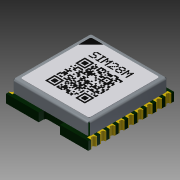
# Autodesk Inventor part: SIM28M
Saved by Autodesk Inventor 2015 SP1 (Build 190203100, 203)
## iProperties
Created: 2015-01-28
Part Number: SIM28M
Material: Типовые
Document SubType Name: Modeling
Designer: Danil
Density: 1 g/cm^3
Appearance: Цинк
Author: Danil
Autodesk Inventor part; units mm, degrees
(part 1 of 2)
ref_plane "YZ Plane" through (0, 0, 0) normal (1, 0, 0) x (0, 1, 0)
sketch "Эскиз1" plane through (0, 0, 0) normal (0, 0, 1) x (1, 0, 0)
  line L0 (4.85, -5.05) -> (-4.85, 5.05) construction
  line L1 (-4.85, -5.05) -> (4.85, 5.05) construction
  line L2 (-1.5, 5.05) -> (-2, 5.05)
  line L3 (1, 4.5) -> (1, 5.05)
  line L4 (-1.5, 5.05) -> (-1.5, 4.5)
  line L5 (-1.25, 4.25) -> (0.75, 4.25)
  line L6 (-4.85, 5.05) -> (-3.85, 5.05)
  line L7 (1, 5.05) -> (1.5, 5.05)
  line L8 (1.5, -5.05) -> (1.5, -4.5)
  line L9 (1.25, -4.25) -> (0, -4.25)
  line L10 (-1, -5.05) -> (-1, -4.5)
  line L11 (-0.75, -4.25) -> (0, -4.25)
  line L12 (4.85, -5.05) -> (1.5, -5.05)
  line L13 (-1, -5.05) -> (-4.85, -5.05)
  arc A0 (0.75, 4.25) -> (1, 4.5) centre (0.75, 4.5) ccw
  arc A1 (-1.5, 4.5) -> (-1.25, 4.25) centre (-1.25, 4.5) ccw
  arc A2 (1.5, -4.5) -> (1.25, -4.25) centre (1.25, -4.5) ccw
  arc A3 (-0.75, -4.25) -> (-1, -4.5) centre (-0.75, -4.5) ccw
  line L14 (4.85, -5.05) -> (1.5, -5.05)
  line L15 (-4.85, 5.05) -> (-1.5, 5.05)
  line L16 (1, 5.05) -> (4.85, 5.05)
  line L17 (-1, -5.05) -> (-4.85, -5.05)
  line L18 (-3.85, 5.05) -> (-1.5, 5.05)
  line L19 (1.5, 5.05) -> (4.85, 5.05)
  line L20 (-1.7057, -5.05) -> (-1, -5.05)
  line L21 (1.5, -5.05) -> (2.7193, -5.05)
  line L22 (-4.85, 1.8825) -> (-4.85, 3.4137)
  arc A4 (-4.85, 4.14) -> (-4.85, 4.66) centre (-4.85, 4.4) ccw
  line L23 (-4.85, 5.05) -> (-4.85, 4.66)
  arc A5 (-4.85, 3.04) -> (-4.85, 3.56) centre (-4.85, 3.3) ccw
  arc A6 (-4.85, 1.94) -> (-4.85, 2.46) centre (-4.85, 2.2) ccw
  arc A7 (-4.85, 0.84) -> (-4.85, 1.36) centre (-4.85, 1.1) ccw
  arc A8 (-4.85, -0.26) -> (-4.85, 0.26) centre (-4.85, 0) ccw
  arc A9 (-4.85, -1.36) -> (-4.85, -0.84) centre (-4.85, -1.1) ccw
  arc A10 (-4.85, -2.46) -> (-4.85, -1.94) centre (-4.85, -2.2) ccw
  arc A11 (-4.85, -3.56) -> (-4.85, -3.04) centre (-4.85, -3.3) ccw
  arc A12 (-4.85, -4.66) -> (-4.85, -4.14) centre (-4.85, -4.4) ccw
  arc A13 (4.85, 4.66) -> (4.85, 4.14) centre (4.85, 4.4) ccw
  arc A14 (4.85, 3.56) -> (4.85, 3.04) centre (4.85, 3.3) ccw
  arc A15 (4.85, 2.46) -> (4.85, 1.94) centre (4.85, 2.2) ccw
  arc A16 (4.85, 1.36) -> (4.85, 0.84) centre (4.85, 1.1) ccw
  arc A17 (4.85, 0.26) -> (4.85, -0.26) centre (4.85, 0) ccw
  arc A18 (4.85, -0.84) -> (4.85, -1.36) centre (4.85, -1.1) ccw
  arc A19 (4.85, -1.94) -> (4.85, -2.46) centre (4.85, -2.2) ccw
  arc A20 (4.85, -3.04) -> (4.85, -3.56) centre (4.85, -3.3) ccw
  arc A21 (4.85, -4.14) -> (4.85, -4.66) centre (4.85, -4.4) ccw
  line L24 (4.85, 5.05) -> (4.85, 4.66)
  line L25 (4.85, 4.14) -> (4.85, 3.56)
  line L26 (4.85, 3.04) -> (4.85, 2.46)
  line L27 (4.85, 1.94) -> (4.85, 1.36)
  line L28 (4.85, 0.84) -> (4.85, 0.26)
  line L29 (4.85, -0.26) -> (4.85, -0.84)
  line L30 (4.85, -1.36) -> (4.85, -1.94)
  line L31 (4.85, -2.46) -> (4.85, -3.04)
  line L32 (4.85, -3.56) -> (4.85, -4.14)
  line L33 (4.85, -4.66) -> (4.85, -5.05)
  line L34 (-4.85, -4.66) -> (-4.85, -5.05)
  line L35 (-4.85, -3.56) -> (-4.85, -4.14)
  line L36 (-4.85, -2.46) -> (-4.85, -3.04)
  line L37 (-4.85, -1.36) -> (-4.85, -1.94)
  line L38 (-4.85, -0.26) -> (-4.85, -0.84)
  line L39 (-4.85, 0.84) -> (-4.85, 0.26)
  line L40 (-4.85, 1.94) -> (-4.85, 1.36)
  line L41 (-4.85, 4.14) -> (-4.85, 3.56)
  line L42 (-4.85, 3.04) -> (-4.85, 2.46)
  point P0 (0, 0)
  point P1 (-4.85, -1.1)
  point P2 (4.85, -1.1)
  dimension "d497" = 1.1
  dimension "d93" = 9.7
  dimension "d98" = 0.25
  dimension "d148" = 0.26
  dimension "d149" = 0.26
  dimension "d150" = 0.26
  dimension "d151" = 0.26
  dimension "d152" = 0.26
  dimension "d153" = 0.26
  dimension "d154" = 0.26
  dimension "d155" = 0.26
  dimension "d156" = 0.26
  dimension "d157" = 0.26
  dimension "d158" = 0.26
  dimension "d159" = 0.26
  dimension "d160" = 0.26
  dimension "d161" = 0.26
  dimension "d162" = 0.26
  dimension "d163" = 0.26
  dimension "d164" = 0.26
  dimension "d165" = 0.26
  constraints: 86 end point, 44 point on circle, 22 centre point, 20 vertical, 12 parallel, 10 perpendicular, 8 tangent, 5 horizontal, 5 point on line, 3 equal radius, 2 coincident, 2 midpoint
  measures "d93" distance of L1.end L0.end
  measures "d98" radius of A0
  measures "d148" radius of A4
  measures "d149" radius of A5
  measures "d150" radius of A6
  measures "d151" radius of A7
  measures "d152" radius of A8
  measures "d153" radius of A9
  measures "d154" radius of A10
  measures "d155" radius of A11
  measures "d156" radius of A12
  measures "d157" radius of A13
  measures "d158" radius of A14
  measures "d159" radius of A15
  measures "d160" radius of A16
  measures "d161" radius of A17
  measures "d162" radius of A18
  measures "d163" radius of A19
  measures "d164" radius of A20
  measures "d165" radius of A21
extrude "Выдавливание2" add sketch "Эскиз1" along normal blind 1 contours L4 A1 L5 A0 L3 L7 L16 L24 A13 L25 A14 L26 A15 L27 A16 L28 A17 L29 A18 L30 A19 L31 A20 L32 A21 L33 L12 L8 A2 L9 L11 A3 L10 L13 L34 A12 L35 A11 L36 A10 L37 A9 L38 A8 L39 A7 L40 L22 A6 A5 L41 A4 L23 L6 L15 L2
sketch "Эскиз4" plane through (0, 0, 0) normal (0, 0, 1) x (1, 0, 0)
  arc A0 (-4.86, 4.15) -> (-4.86, 4.65) centre (-4.86, 4.4) ccw
  line L0 (-4.86, 4.4) -> (-4.86, 4.65) construction
  line L1 (-4.86, 4.4) -> (-4.61, 4.4) construction
  line L2 (-4.86, 4.4) -> (-4.86, 4.15) construction
  line L3 (-4.86, 4.65) -> (-4.86, 4.75)
  line L4 (-4.86, 4.65) -> (-4.76, 4.65) construction
  line L5 (-4.86, 4.75) -> (-4.41, 4.75)
  line L6 (-4.41, 4.75) -> (-4.41, 4.05)
  line L7 (-4.41, 4.05) -> (-4.86, 4.05)
  line L8 (-4.86, 4.05) -> (-4.86, 4.15)
  arc A1 (4.86, 4.65) -> (4.86, 4.15) centre (4.86, 4.4) ccw
  line L9 (4.86, 4.4) -> (4.86, 4.65) construction
  line L10 (4.86, 4.4) -> (5.11, 4.4) construction
  line L11 (4.86, 4.4) -> (4.86, 4.15) construction
  line L12 (4.86, 4.65) -> (4.86, 4.75)
  line L13 (4.86, 4.75) -> (4.41, 4.75)
  line L14 (4.41, 4.75) -> (4.41, 4.05)
  line L15 (4.41, 4.05) -> (4.86, 4.05)
  line L16 (4.86, 4.05) -> (4.86, 4.15)
  line L17 (4.86, 3.3) -> (4.86, 3.55) construction
  arc A2 (4.86, 3.55) -> (4.86, 3.05) centre (4.86, 3.3) ccw
  line L18 (4.86, 3.55) -> (4.86, 3.65)
  line L19 (4.86, 3.65) -> (4.41, 3.65)
  line L20 (4.41, 3.65) -> (4.41, 2.95)
  line L21 (4.41, 2.95) -> (4.86, 2.95)
  line L22 (4.86, 2.95) -> (4.86, 3.05)
  line L23 (4.86, 1.85) -> (4.86, 1.95)
  line L24 (4.41, 2.55) -> (4.41, 1.85)
  line L25 (4.86, 2.2) -> (4.86, 2.45) construction
  arc A3 (4.86, 2.45) -> (4.86, 1.95) centre (4.86, 2.2) ccw
  line L26 (4.86, 2.45) -> (4.86, 2.55)
  line L27 (4.86, 2.55) -> (4.41, 2.55)
  line L28 (4.41, 1.85) -> (4.86, 1.85)
  line L29 (4.86, 0.75) -> (4.86, 0.85)
  line L30 (4.41, 1.45) -> (4.41, 0.75)
  line L31 (4.86, 1.1) -> (4.86, 1.35) construction
  arc A4 (4.86, 1.35) -> (4.86, 0.85) centre (4.86, 1.1) ccw
  line L32 (4.86, 1.35) -> (4.86, 1.45)
  line L33 (4.86, 1.45) -> (4.41, 1.45)
  line L34 (4.41, 0.75) -> (4.86, 0.75)
  line L35 (4.86, -0.35) -> (4.86, -0.25)
  line L36 (4.41, 0.35) -> (4.41, -0.35)
  line L37 (4.86, 0) -> (4.86, 0.25) construction
  arc A5 (4.86, 0.25) -> (4.86, -0.25) centre (4.86, 0) ccw
  line L38 (4.86, 0.25) -> (4.86, 0.35)
  line L39 (4.86, 0.35) -> (4.41, 0.35)
  line L40 (4.41, -0.35) -> (4.86, -0.35)
  line L41 (4.86, -1.45) -> (4.86, -1.35)
  line L42 (4.41, -0.75) -> (4.41, -1.45)
  line L43 (4.86, -1.1) -> (4.86, -0.85) construction
  arc A6 (4.86, -0.85) -> (4.86, -1.35) centre (4.86, -1.1) ccw
  line L44 (4.86, -0.85) -> (4.86, -0.75)
  line L45 (4.86, -0.75) -> (4.41, -0.75)
  line L46 (4.41, -1.45) -> (4.86, -1.45)
  line L47 (4.86, -2.55) -> (4.86, -2.45)
  line L48 (4.41, -1.85) -> (4.41, -2.55)
  line L49 (4.86, -2.2) -> (4.86, -1.95) construction
  arc A7 (4.86, -1.95) -> (4.86, -2.45) centre (4.86, -2.2) ccw
  line L50 (4.86, -1.95) -> (4.86, -1.85)
  line L51 (4.86, -1.85) -> (4.41, -1.85)
  line L52 (4.41, -2.55) -> (4.86, -2.55)
  line L53 (4.86, -3.65) -> (4.86, -3.55)
  line L54 (4.41, -2.95) -> (4.41, -3.65)
  line L55 (4.86, -3.3) -> (4.86, -3.05) construction
  arc A8 (4.86, -3.05) -> (4.86, -3.55) centre (4.86, -3.3) ccw
  line L56 (4.86, -3.05) -> (4.86, -2.95)
  line L57 (4.86, -2.95) -> (4.41, -2.95)
  line L58 (4.41, -3.65) -> (4.86, -3.65)
  line L59 (4.86, -4.75) -> (4.86, -4.65)
  line L60 (4.41, -4.05) -> (4.41, -4.75)
  line L61 (4.86, -4.4) -> (4.86, -4.15) construction
  arc A9 (4.86, -4.15) -> (4.86, -4.65) centre (4.86, -4.4) ccw
  line L62 (4.86, -4.15) -> (4.86, -4.05)
  line L63 (4.86, -4.05) -> (4.41, -4.05)
  line L64 (4.41, -4.75) -> (4.86, -4.75)
  arc A10 (-4.86, 3.05) -> (-4.86, 3.55) centre (-4.86, 3.3) ccw
  line L65 (-4.86, 3.3) -> (-4.61, 3.3) construction
  line L66 (-4.86, 3.65) -> (-4.41, 3.65)
  line L67 (-4.41, 3.65) -> (-4.41, 2.95)
  line L68 (-4.41, 2.95) -> (-4.86, 2.95)
  line L69 (-4.86, 3.55) -> (-4.86, 3.65)
  line L70 (-4.86, 2.95) -> (-4.86, 3.05)
  line L71 (-4.86, 2.55) -> (-4.41, 2.55)
  line L72 (-4.86, 2.2) -> (-4.61, 2.2) construction
  arc A11 (-4.86, 1.95) -> (-4.86, 2.45) centre (-4.86, 2.2) ccw
  line L73 (-4.41, 1.85) -> (-4.86, 1.85)
  line L74 (-4.41, 2.55) -> (-4.41, 1.85)
  line L75 (-4.86, 2.45) -> (-4.86, 2.55)
  line L76 (-4.86, 1.85) -> (-4.86, 1.95)
  line L77 (-4.86, 1.45) -> (-4.41, 1.45)
  line L78 (-4.86, 1.1) -> (-4.61, 1.1) construction
  arc A12 (-4.86, 0.85) -> (-4.86, 1.35) centre (-4.86, 1.1) ccw
  line L79 (-4.41, 0.75) -> (-4.86, 0.75)
  line L80 (-4.41, 1.45) -> (-4.41, 0.75)
  line L81 (-4.86, 1.35) -> (-4.86, 1.45)
  line L82 (-4.86, 0.75) -> (-4.86, 0.85)
  line L83 (-4.86, 0.35) -> (-4.41, 0.35)
  line L84 (-4.86, 0) -> (-4.61, 0) construction
  arc A13 (-4.86, -0.25) -> (-4.86, 0.25) centre (-4.86, 0) ccw
  line L85 (-4.41, -0.35) -> (-4.86, -0.35)
  line L86 (-4.41, 0.35) -> (-4.41, -0.35)
  line L87 (-4.86, 0.25) -> (-4.86, 0.35)
  line L88 (-4.86, -0.35) -> (-4.86, -0.25)
  line L89 (-4.86, -0.75) -> (-4.41, -0.75)
  line L90 (-4.86, -1.1) -> (-4.61, -1.1) construction
  arc A14 (-4.86, -1.35) -> (-4.86, -0.85) centre (-4.86, -1.1) ccw
  line L91 (-4.41, -1.45) -> (-4.86, -1.45)
  line L92 (-4.41, -0.75) -> (-4.41, -1.45)
  line L93 (-4.86, -0.85) -> (-4.86, -0.75)
  line L94 (-4.86, -1.45) -> (-4.86, -1.35)
  line L95 (-4.86, -1.85) -> (-4.41, -1.85)
  line L96 (-4.86, -2.2) -> (-4.61, -2.2) construction
  arc A15 (-4.86, -2.45) -> (-4.86, -1.95) centre (-4.86, -2.2) ccw
  line L97 (-4.41, -2.55) -> (-4.86, -2.55)
  line L98 (-4.41, -1.85) -> (-4.41, -2.55)
  line L99 (-4.86, -1.95) -> (-4.86, -1.85)
  line L100 (-4.86, -2.55) -> (-4.86, -2.45)
  line L101 (-4.86, -2.95) -> (-4.41, -2.95)
  line L102 (-4.86, -3.3) -> (-4.61, -3.3) construction
  arc A16 (-4.86, -3.55) -> (-4.86, -3.05) centre (-4.86, -3.3) ccw
  line L103 (-4.41, -3.65) -> (-4.86, -3.65)
  line L104 (-4.41, -2.95) -> (-4.41, -3.65)
  line L105 (-4.86, -3.05) -> (-4.86, -2.95)
  line L106 (-4.86, -3.65) -> (-4.86, -3.55)
  line L107 (-4.86, -4.05) -> (-4.41, -4.05)
  line L108 (-4.86, -4.4) -> (-4.61, -4.4) construction
  arc A17 (-4.86, -4.65) -> (-4.86, -4.15) centre (-4.86, -4.4) ccw
  line L109 (-4.41, -4.75) -> (-4.86, -4.75)
  line L110 (-4.41, -4.05) -> (-4.41, -4.75)
  line L111 (-4.86, -4.15) -> (-4.86, -4.05)
  line L112 (-4.86, -4.75) -> (-4.86, -4.65)
  point P0 (-4.86, 0)
  point P1 (-4.86, -2.2)
  point P2 (-4.86, -3.3)
  point P3 (4.86, -2.2)
  point P4 (4.86, -3.3)
  point P5 (-4.86, -4.4)
  dimension "d354" = 0.25
  dimension "d355" = 90
  dimension "d356" = 180
  dimension "d357" = 0.1
  dimension "d358" = 90
  dimension "d359" = 0.45
  dimension "d360" = 0.7
  dimension "d361" = 0.25
  dimension "d362" = 90
  dimension "d363" = 180
  dimension "d364" = 0.1
  dimension "d365" = 0.45
  dimension "d366" = 0.7
  dimension "d367" = 0.25
  dimension "d368" = 0.1
  dimension "d369" = 0.45
  dimension "d370" = 0.7
  dimension "d371" = 0.25
  dimension "d372" = 0.1
  dimension "d373" = 0.45
  dimension "d374" = 0.7
  dimension "d375" = 0.25
  dimension "d376" = 0.1
  dimension "d377" = 0.45
  dimension "d378" = 0.7
  dimension "d379" = 0.25
  dimension "d380" = 0.1
  dimension "d381" = 0.45
  dimension "d382" = 0.7
  dimension "d383" = 0.25
  dimension "d384" = 0.1
  dimension "d385" = 0.45
  dimension "d386" = 0.7
  dimension "d387" = 0.25
  dimension "d388" = 0.1
  dimension "d389" = 0.45
  dimension "d390" = 0.7
  dimension "d391" = 0.25
  dimension "d392" = 0.1
  dimension "d393" = 0.45
  dimension "d394" = 0.7
  dimension "d395" = 0.25
  dimension "d396" = 0.1
  dimension "d397" = 0.45
  dimension "d398" = 0.7
  dimension "d399" = 0.25
  dimension "d400" = 0.1
  dimension "d401" = 0.45
  dimension "d402" = 0.7
  dimension "d403" = 0.25
  dimension "d404" = 0.1
  dimension "d405" = 0.45
  dimension "d406" = 0.7
  dimension "d407" = 0.25
  dimension "d408" = 0.1
  dimension "d409" = 0.45
  dimension "d410" = 0.7
  dimension "d411" = 0.25
  dimension "d412" = 0.1
  dimension "d413" = 0.45
  dimension "d414" = 0.7
  dimension "d415" = 0.25
  dimension "d416" = 0.1
  dimension "d417" = 0.45
  constraints: 226 end point, 57 perpendicular, 36 point on circle, 29 horizontal, 18 centre point, 18 vertical, 2 coincident
  measures "d354" radius of A0
  measures "d355" angle of L1 L0
  measures "d356" angle of L0 L2
  measures "d357" distance of L0.end L3.end
  measures "d358" angle of L4 L3
  measures "d359" distance of L3.end L5.end
  measures "d360" distance of L5.end L6.end
  measures "d361" radius of A1
  measures "d362" angle of L10 L9
  measures "d363" angle of L9 L11
  measures "d364" distance of L9.end L12.end
  measures "d365" distance of L12.end L13.end
  measures "d366" distance of L13.end L14.end
  measures "d367" radius of A2
  measures "d368" distance of L17.end L18.end
  measures "d369" distance of L18.end L19.end
  measures "d370" distance of L19.end L20.end
  measures "d371" radius of A3
  measures "d372" distance of L25.end L26.end
  measures "d373" distance of L26.end L24.start
  measures "d374" distance of L24.start L24.end
  measures "d375" radius of A4
  measures "d376" distance of L31.end L32.end
  measures "d377" distance of L32.end L30.start
  measures "d378" distance of L30.start L30.end
  measures "d379" radius of A5
  measures "d380" distance of L37.end L38.end
  measures "d381" distance of L38.end L36.start
  measures "d382" distance of L36.start L36.end
  measures "d383" radius of A6
  measures "d384" distance of L43.end L44.end
  measures "d385" distance of L44.end L42.start
  measures "d386" distance of L42.start L42.end
  measures "d387" radius of A7
  measures "d388" distance of L49.end L50.end
  measures "d389" distance of L50.end L48.start
  measures "d390" distance of L48.start L48.end
  measures "d391" radius of A8
  measures "d392" distance of L55.end L56.end
  measures "d393" distance of L56.end L54.start
  measures "d394" distance of L54.start L54.end
  measures "d395" radius of A9
  measures "d396" distance of L61.end L62.end
  measures "d397" distance of L62.end L60.start
  measures "d398" distance of L60.start L60.end
  measures "d399" radius of A10
  measures "d400" distance of L69.start L66.start
  measures "d401" distance of L66.start L66.end
  measures "d402" distance of L66.end L67.end
  measures "d403" radius of A11
  measures "d404" distance of L75.start L71.start
  measures "d405" distance of L71.start L71.end
  measures "d406" distance of L71.end L73.start
  measures "d407" radius of A12
  measures "d408" distance of L81.start L77.start
  measures "d409" distance of L77.start L77.end
  measures "d410" distance of L77.end L79.start
  measures "d411" radius of A13
  measures "d412" distance of L87.start L83.start
  measures "d413" distance of L83.start L83.end
  measures "d414" distance of L83.end L85.start
  measures "d415" radius of A14
  measures "d416" distance of L93.start L89.start
  measures "d417" distance of L89.start L89.end
extrude "Выдавливание3" add sketch "Эскиз4" along normal blind 1.01
sketch "Эскиз2" plane through (0, 0, 0) normal (0, 0, 1) x (1, 0, 0)
  arc A0 (-4.86, 4.15) -> (-4.86, 4.65) centre (-4.86, 4.4) ccw
  line L0 (-4.86, 4.4) -> (-4.86, 4.65) construction
  line L1 (-4.86, 4.4) -> (-4.61, 4.4) construction
  line L2 (-4.86, 4.4) -> (-4.86, 4.15) construction
  line L3 (-4.86, 4.65) -> (-4.86, 4.75)
  line L4 (-4.86, 4.65) -> (-4.76, 4.65) construction
  line L5 (-4.86, 4.75) -> (-3.86, 4.75)
  line L6 (-3.86, 4.75) -> (-3.86, 4.05)
  line L7 (-3.86, 4.05) -> (-4.86, 4.05)
  line L8 (-4.86, 4.05) -> (-4.86, 4.15)
  arc A1 (4.86, 4.65) -> (4.86, 4.15) centre (4.86, 4.4) ccw
  line L9 (4.86, 4.4) -> (4.86, 4.65) construction
  line L10 (4.86, 4.4) -> (5.11, 4.4) construction
  line L11 (4.86, 4.4) -> (4.86, 4.15) construction
  line L12 (4.86, 4.65) -> (4.86, 4.75)
  line L13 (4.86, 4.75) -> (3.86, 4.75)
  line L14 (3.86, 4.75) -> (3.86, 4.05)
  line L15 (3.86, 4.05) -> (4.86, 4.05)
  line L16 (4.86, 4.05) -> (4.86, 4.15)
  arc A2 (4.86, 3.55) -> (4.86, 3.05) centre (4.86, 3.3) ccw
  line L17 (4.86, 3.3) -> (4.86, 3.55) construction
  line L18 (4.86, 3.55) -> (4.86, 3.65)
  line L19 (4.86, 3.65) -> (3.86, 3.65)
  line L20 (3.86, 3.65) -> (3.86, 2.95)
  line L21 (3.86, 2.95) -> (4.86, 2.95)
  line L22 (4.86, 2.95) -> (4.86, 3.05)
  line L23 (4.86, 2.2) -> (4.86, 2.45) construction
  arc A3 (4.86, 2.45) -> (4.86, 1.95) centre (4.86, 2.2) ccw
  line L24 (4.86, 2.45) -> (4.86, 2.55)
  line L25 (4.86, 2.55) -> (3.86, 2.55)
  line L26 (3.86, 2.55) -> (3.86, 1.85)
  line L27 (3.86, 1.85) -> (4.86, 1.85)
  line L28 (4.86, 1.85) -> (4.86, 1.95)
  line L29 (4.86, 1.1) -> (4.86, 1.35) construction
  arc A4 (4.86, 1.35) -> (4.86, 0.85) centre (4.86, 1.1) ccw
  line L30 (4.86, 1.35) -> (4.86, 1.45)
  line L31 (4.86, 1.45) -> (3.86, 1.45)
  line L32 (3.86, 1.45) -> (3.86, 0.75)
  line L33 (3.86, 0.75) -> (4.86, 0.75)
  line L34 (4.86, 0.75) -> (4.86, 0.85)
  line L35 (4.86, 0) -> (4.86, 0.25) construction
  arc A5 (4.86, 0.25) -> (4.86, -0.25) centre (4.86, 0) ccw
  line L36 (4.86, 0.25) -> (4.86, 0.35)
  line L37 (4.86, 0.35) -> (3.86, 0.35)
  line L38 (3.86, 0.35) -> (3.86, -0.35)
  line L39 (3.86, -0.35) -> (4.86, -0.35)
  line L40 (4.86, -0.35) -> (4.86, -0.25)
  line L41 (4.86, -1.1) -> (4.86, -0.85) construction
  arc A6 (4.86, -0.85) -> (4.86, -1.35) centre (4.86, -1.1) ccw
  line L42 (4.86, -0.85) -> (4.86, -0.75)
  line L43 (4.86, -0.75) -> (3.86, -0.75)
  line L44 (3.86, -0.75) -> (3.86, -1.45)
  line L45 (3.86, -1.45) -> (4.86, -1.45)
  line L46 (4.86, -1.45) -> (4.86, -1.35)
  line L47 (4.86, -2.2) -> (4.86, -1.95) construction
  arc A7 (4.86, -1.95) -> (4.86, -2.45) centre (4.86, -2.2) ccw
  line L48 (4.86, -1.95) -> (4.86, -1.85)
  line L49 (4.86, -1.85) -> (3.86, -1.85)
  line L50 (3.86, -1.85) -> (3.86, -2.55)
  line L51 (3.86, -2.55) -> (4.86, -2.55)
  line L52 (4.86, -2.55) -> (4.86, -2.45)
  line L53 (4.86, -3.3) -> (4.86, -3.05) construction
  arc A8 (4.86, -3.05) -> (4.86, -3.55) centre (4.86, -3.3) ccw
  line L54 (4.86, -3.05) -> (4.86, -2.95)
  line L55 (4.86, -2.95) -> (3.86, -2.95)
  line L56 (3.86, -2.95) -> (3.86, -3.65)
  line L57 (3.86, -3.65) -> (4.86, -3.65)
  line L58 (4.86, -3.65) -> (4.86, -3.55)
  line L59 (4.86, -4.4) -> (4.86, -4.15) construction
  arc A9 (4.86, -4.15) -> (4.86, -4.65) centre (4.86, -4.4) ccw
  line L60 (4.86, -4.15) -> (4.86, -4.05)
  line L61 (4.86, -4.05) -> (3.86, -4.05)
  line L62 (3.86, -4.05) -> (3.86, -4.75)
  line L63 (3.86, -4.75) -> (4.86, -4.75)
  line L64 (4.86, -4.75) -> (4.86, -4.65)
  arc A10 (-4.86, 3.05) -> (-4.86, 3.55) centre (-4.86, 3.3) ccw
  line L65 (-4.86, 3.3) -> (-4.61, 3.3) construction
  line L66 (-4.86, 3.55) -> (-4.86, 3.65)
  line L67 (-4.86, 3.65) -> (-3.86, 3.65)
  line L68 (-3.86, 3.65) -> (-3.86, 2.95)
  line L69 (-3.86, 2.95) -> (-4.86, 2.95)
  line L70 (-4.86, 2.95) -> (-4.86, 3.05)
  arc A11 (-4.86, 1.95) -> (-4.86, 2.45) centre (-4.86, 2.2) ccw
  line L71 (-4.86, 2.2) -> (-4.61, 2.2) construction
  line L72 (-4.86, 2.55) -> (-3.86, 2.55)
  line L73 (-3.86, 2.55) -> (-3.86, 1.85)
  line L74 (-3.86, 1.85) -> (-4.86, 1.85)
  line L75 (-4.86, 2.45) -> (-4.86, 2.55)
  line L76 (-4.86, 1.85) -> (-4.86, 1.95)
  arc A12 (-4.86, 0.85) -> (-4.86, 1.35) centre (-4.86, 1.1) ccw
  line L77 (-4.86, 1.1) -> (-4.61, 1.1) construction
  line L78 (-4.86, 1.45) -> (-3.86, 1.45)
  line L79 (-3.86, 1.45) -> (-3.86, 0.75)
  line L80 (-3.86, 0.75) -> (-4.86, 0.75)
  line L81 (-4.86, 1.35) -> (-4.86, 1.45)
  line L82 (-4.86, 0.75) -> (-4.86, 0.85)
  arc A13 (-4.86, -0.25) -> (-4.86, 0.25) centre (-4.86, 0) ccw
  line L83 (-4.86, 0) -> (-4.61, 0) construction
  line L84 (-4.86, 0.35) -> (-3.86, 0.35)
  line L85 (-3.86, 0.35) -> (-3.86, -0.35)
  line L86 (-3.86, -0.35) -> (-4.86, -0.35)
  line L87 (-4.86, 0.25) -> (-4.86, 0.35)
  line L88 (-4.86, -0.35) -> (-4.86, -0.25)
  arc A14 (-4.86, -1.35) -> (-4.86, -0.85) centre (-4.86, -1.1) ccw
  line L89 (-4.86, -1.1) -> (-4.61, -1.1) construction
  line L90 (-4.86, -0.75) -> (-3.86, -0.75)
  line L91 (-3.86, -0.75) -> (-3.86, -1.45)
  line L92 (-3.86, -1.45) -> (-4.86, -1.45)
  line L93 (-4.86, -0.85) -> (-4.86, -0.75)
  line L94 (-4.86, -1.45) -> (-4.86, -1.35)
  arc A15 (-4.86, -2.45) -> (-4.86, -1.95) centre (-4.86, -2.2) ccw
  line L95 (-4.86, -2.2) -> (-4.61, -2.2) construction
  line L96 (-4.86, -1.85) -> (-3.86, -1.85)
  line L97 (-3.86, -1.85) -> (-3.86, -2.55)
  line L98 (-3.86, -2.55) -> (-4.86, -2.55)
  line L99 (-4.86, -1.95) -> (-4.86, -1.85)
  line L100 (-4.86, -2.55) -> (-4.86, -2.45)
  arc A16 (-4.86, -3.55) -> (-4.86, -3.05) centre (-4.86, -3.3) ccw
  line L101 (-4.86, -3.3) -> (-4.61, -3.3) construction
  line L102 (-4.86, -2.95) -> (-3.86, -2.95)
  line L103 (-3.86, -2.95) -> (-3.86, -3.65)
  line L104 (-3.86, -3.65) -> (-4.86, -3.65)
  line L105 (-4.86, -3.05) -> (-4.86, -2.95)
  line L106 (-4.86, -3.65) -> (-4.86, -3.55)
  arc A17 (-4.86, -4.65) -> (-4.86, -4.15) centre (-4.86, -4.4) ccw
  line L107 (-4.86, -4.4) -> (-4.61, -4.4) construction
  line L108 (-4.86, -4.05) -> (-3.86, -4.05)
  line L109 (-3.86, -4.05) -> (-3.86, -4.75)
  line L110 (-3.86, -4.75) -> (-4.86, -4.75)
  line L111 (-4.86, -4.15) -> (-4.86, -4.05)
  line L112 (-4.86, -4.75) -> (-4.86, -4.65)
  point P0 (-4.86, 0)
  point P1 (-4.86, -2.2)
  point P2 (-4.86, -3.3)
  point P3 (4.86, 2.2)
  point P4 (4.86, -2.2)
  point P5 (4.86, -3.3)
  point P6 (4.86, 4.4)
  dimension "d188" = 0.25
  dimension "d189" = 90
  dimension "d190" = 180
  dimension "d191" = 0.1
  dimension "d192" = 90
  dimension "d193" = 1
  dimension "d194" = 0.7
  dimension "d227" = 0.25
  dimension "d228" = 90
  dimension "d229" = 180
  dimension "d230" = 0.1
  dimension "d231" = 1
  dimension "d232" = 0.7
  dimension "d233" = 0.25
  dimension "d234" = 0.1
  dimension "d235" = 1
  dimension "d236" = 0.7
  dimension "d237" = 0.25
  dimension "d238" = 0.1
  dimension "d239" = 1
  dimension "d240" = 0.7
  dimension "d245" = 0.25
  dimension "d246" = 0.1
  dimension "d247" = 1
  dimension "d248" = 0.7
  dimension "d253" = 0.25
  dimension "d254" = 0.1
  dimension "d255" = 1
  dimension "d256" = 0.7
  dimension "d261" = 0.25
  dimension "d262" = 0.1
  dimension "d263" = 1
  dimension "d264" = 0.7
  dimension "d269" = 0.25
  dimension "d270" = 0.1
  dimension "d271" = 1
  dimension "d272" = 0.7
  dimension "d277" = 0.25
  dimension "d278" = 0.1
  dimension "d279" = 1
  dimension "d280" = 0.7
  dimension "d285" = 0.25
  dimension "d286" = 0.1
  dimension "d287" = 1
  dimension "d288" = 0.7
  dimension "d293" = 0.25
  dimension "d294" = 0.1
  dimension "d296" = 1
  dimension "d297" = 0.7
  dimension "d298" = 0.25
  dimension "d299" = 0.1
  dimension "d300" = 1
  dimension "d301" = 0.7
  dimension "d306" = 0.25
  dimension "d307" = 0.1
  dimension "d308" = 1
  dimension "d309" = 0.7
  dimension "d314" = 0.25
  dimension "d315" = 0.1
  dimension "d316" = 1
  dimension "d317" = 0.7
  dimension "d322" = 0.25
  dimension "d323" = 0.1
  dimension "d324" = 1
  constraints: 226 end point, 57 perpendicular, 36 point on circle, 29 horizontal, 18 centre point, 18 vertical, 2 coincident
  measures "d188" radius of A0
  measures "d189" angle of L1 L0
  measures "d190" angle of L0 L2
  measures "d191" distance of L0.end L3.end
  measures "d192" angle of L4 L3
  measures "d193" distance of L3.end L5.end
  measures "d194" distance of L5.end L6.end
  measures "d227" radius of A1
  measures "d228" angle of L10 L9
  measures "d229" angle of L9 L11
  measures "d230" distance of L9.end L12.end
  measures "d231" distance of L12.end L13.end
  measures "d232" distance of L13.end L14.end
  measures "d233" radius of A2
  measures "d234" distance of L17.end L18.end
  measures "d235" distance of L18.end L19.end
  measures "d236" distance of L19.end L20.end
  measures "d237" radius of A3
  measures "d238" distance of L23.end L24.end
  measures "d239" distance of L24.end L26.start
  measures "d240" distance of L26.start L26.end
  measures "d245" radius of A4
  measures "d246" distance of L29.end L30.end
  measures "d247" distance of L30.end L32.start
  measures "d248" distance of L32.start L32.end
  measures "d253" radius of A5
  measures "d254" distance of L35.end L36.end
  measures "d255" distance of L36.end L38.start
  measures "d256" distance of L38.start L38.end
  measures "d261" radius of A6
  measures "d262" distance of L41.end L42.end
  measures "d263" distance of L42.end L44.start
  measures "d264" distance of L44.start L44.end
  measures "d269" radius of A7
  measures "d270" distance of L47.end L48.end
  measures "d271" distance of L48.end L50.start
  measures "d272" distance of L50.start L50.end
  measures "d277" radius of A8
  measures "d278" distance of L53.end L54.end
  measures "d279" distance of L54.end L56.start
  measures "d280" distance of L56.start L56.end
  measures "d285" radius of A9
  measures "d286" distance of L59.end L60.end
  measures "d287" distance of L60.end L62.start
  measures "d288" distance of L62.start L62.end
  measures "d293" radius of A10
  measures "d294" distance of L66.start L67.start
  measures "d296" distance of L67.start L67.end
  measures "d297" distance of L67.end L68.end
  measures "d298" radius of A11
  measures "d299" distance of L75.start L72.start
  measures "d300" distance of L72.start L72.end
  measures "d301" distance of L72.end L74.start
  measures "d306" radius of A12
  measures "d307" distance of L81.start L78.start
  measures "d308" distance of L78.start L78.end
  measures "d309" distance of L78.end L80.start
  measures "d314" radius of A13
  measures "d315" distance of L87.start L84.start
  measures "d316" distance of L84.start L84.end
  measures "d317" distance of L84.end L86.start
  measures "d322" radius of A14
  measures "d323" distance of L93.start L90.start
  measures "d324" distance of L90.start L90.end
extrude "Выдавливание4" add sketch "Эскиз2" against normal blind 0.01
ref_plane "РабПлоскость1" through (0, 0, 1.1) normal (0, 0, 1) x (1, 0, 0)
sketch "Эскиз5" plane through (0, 0, 1.1) normal (0, 0, 1) x (1, 0, 0)
  line L0 (-4.55, 4.66) -> (4.55, 4.66)
  line L1 (4.55, 4.66) -> (4.55, -4.66)
  line L2 (4.55, -4.66) -> (-4.55, -4.66)
  line L3 (-4.55, -4.66) -> (-4.55, 4.66)
  line L4 (-4.55, 4.66) -> (-4.35, 4.66)
  line L5 (-4.35, 4.66) -> (-4.35, 4.46)
  line L6 (-4.35, 4.46) -> (-4.55, 4.46)
  line L7 (-4.55, 4.46) -> (-4.55, 4.66)
  line L8 (4.55, 4.66) -> (4.35, 4.66)
  line L9 (4.35, 4.66) -> (4.35, 4.46)
  line L10 (4.35, 4.46) -> (4.55, 4.46)
  line L11 (4.55, 4.46) -> (4.55, 4.66)
  line L12 (-4.55, -4.66) -> (-4.35, -4.66)
  line L13 (-4.35, -4.66) -> (-4.35, -4.46)
  line L14 (-4.35, -4.46) -> (-4.55, -4.46)
  line L15 (-4.55, -4.46) -> (-4.55, -4.66)
  line L16 (4.55, -4.66) -> (4.35, -4.66)
  line L17 (4.35, -4.66) -> (4.35, -4.46)
  line L18 (4.35, -4.46) -> (4.55, -4.46)
  line L19 (4.55, -4.46) -> (4.55, -4.66)
  line L20 (-4.35, -4.46) -> (4.35, -4.46)
  line L21 (4.35, -4.46) -> (4.35, 4.46)
  line L22 (4.35, 4.46) -> (-4.35, 4.46)
  line L23 (-4.35, 4.46) -> (-4.35, -4.46)
  line L24 (-4.45, -4.56) -> (4.45, -4.56)
  line L25 (4.45, -4.56) -> (4.45, 4.56)
  line L26 (4.45, 4.56) -> (-4.45, 4.56)
  line L27 (-4.45, 4.56) -> (-4.45, -4.56)
  dimension "d497" = 1.1
  dimension "d520" = 0.2
  dimension "d521" = 0.2
  dimension "d522" = 0.2
  dimension "d523" = 0.2
  dimension "d524" = 0.2
  dimension "d525" = 0.2
  dimension "d526" = 0.2
  dimension "d527" = 0.2
  constraints: 56 end point, 14 parallel, 7 horizontal, 7 perpendicular
  measures "d520" distance of L5.end L6.end
  measures "d521" distance of L4.end L5.end
  measures "d522" distance of L10.end L9.end
  measures "d523" distance of L9.end L8.end
  measures "d524" distance of L14.end L13.end
  measures "d525" distance of L13.end L12.end
  measures "d526" distance of L17.end L18.end
  measures "d527" distance of L16.end L17.end
extrude "Выдавливание5" add sketch "Эскиз5" along normal blind 1.4 contours L0 L9 L26 L5 | L6 L27 L14 L3 | L26 L9 L22 L5 | L5 L6 L27 L26 | L6 L23 L14 L27 | L26 L25 L10 L9 | L22 L21 L20 L23 | L14 L13 L24 L27 | L1 L18 L25 L10 | L10 L25 L18 L21 | L20 L17 L24 L13 | L13 L24 L17 L2 | L18 L25 L24 L17
extrude "Выдавливание6" cut sketch "Эскиз5" along normal blind 1.3 contours L26 L9 L22 L5 | L5 L6 L27 L26 | L6 L23 L14 L27 | L26 L25 L10 L9 | L22 L21 L20 L23 | L14 L13 L24 L27 | L10 L25 L18 L21 | L20 L17 L24 L13 | L18 L25 L24 L17
fillet "Сопряжение2" radius 0.1 4 edges at (4.45, 0, 2.4) (0, 4.56, 2.4) (-4.45, 0, 2.4) (0, -4.56, 2.4)
sketch "Эскиз8" plane through (0, 0, 0) normal (0, 0, 1) x (1, 0, 0)
  line L0 (1, 4.5) -> (1, 5.05) construction
  line L1 (-1.5, 5.05) -> (-1.5, 4.5) construction
  line L2 (-1.25, 4.25) -> (0.75, 4.25) construction
  line L3 (1.5, -5.05) -> (1.5, -4.5) construction
  line L4 (-1, -5.05) -> (-1, -4.5) construction
  arc A0 (0.75, 4.25) -> (1, 4.5) centre (0.75, 4.5) ccw construction
  arc A1 (-1.5, 4.5) -> (-1.25, 4.25) centre (-1.25, 4.5) ccw construction
  arc A2 (1.5, -4.5) -> (1.25, -4.25) centre (1.25, -4.5) ccw construction
  line L5 (1.2, 4.75) -> (1.2, 4.5)
  arc A3 (0.75, 4.05) -> (1.2, 4.5) centre (0.75, 4.5) ccw
  line L6 (0.75, 4.05) -> (-1.25, 4.05)
  arc A4 (-1.7, 4.5) -> (-1.25, 4.05) centre (-1.25, 4.5) ccw
  line L7 (-1.7, 4.5) -> (-1.7, 4.75)
  line L8 (1.25, -4.25) -> (-0.75, -4.25) construction
  arc A5 (-0.75, -4.25) -> (-1, -4.5) centre (-0.75, -4.5) ccw construction
  line L9 (-1.2, -4.765) -> (-1.2, -4.5)
  arc A6 (-0.75, -4.05) -> (-1.2, -4.5) centre (-0.75, -4.5) ccw
  line L10 (-0.75, -4.05) -> (1.25, -4.05)
  arc A7 (1.7, -4.5) -> (1.25, -4.05) centre (1.25, -4.5) ccw
  line L11 (1.7, -4.5) -> (1.7, -4.75)
  line L12 (-3.882, 4.75) -> (-1.7, 4.75)
  line L13 (-3.882, 4.05) -> (-3.6743, 4.05)
  line L14 (-3.6743, 4.05) -> (-3.6743, -4.765)
  line L15 (-3.882, 4.75) -> (-3.882, 4.05)
  line L16 (3.7043, 4.75) -> (3.7043, -4.05)
  line L17 (3.7043, -4.75) -> (1.7, -4.75)
  line L18 (-1.2, -4.765) -> (-3.6743, -4.765)
  line L19 (1.2, 4.75) -> (3.7043, 4.75)
  line L20 (3.7043, -4.75) -> (3.86, -4.75)
  line L21 (3.86, -4.75) -> (3.86, -4.05)
  line L22 (3.86, -4.05) -> (3.86, -4.75) projected
  line L23 (3.86, -4.05) -> (3.7043, -4.05)
  point P0 (0, 0)
  point P1 (-3.86, 4.05)
  point P2 (-3.86, 4.75)
  dimension "d599" = 0.2
  dimension "d602" = 0.25
  dimension "d603" = 0.2
  constraints: 46 end point, 16 point on circle, 8 centre point, 7 tangent, 5 horizontal alignment, 4 perpendicular, 3 horizontal, 2 equal radius, 2 vertical, 1 collinear, 4 other
  measures "d599" distance between parallel lines of L2 L6
  measures "d602" radius of A5
  measures "d603" distance between parallel lines of L8 L10
extrude "Выдавливание9" cut sketch "Эскиз8" along normal blind 0.01
extrude "Выдавливание11" cut sketch "Эскиз5" along normal blind 1.4 contours L0 L5 L26 L27 L6 L3 | L0 L1 L10 L25 L26 L9 | L5 L6 L27 L26 | L14 L27 L24 L13 L2 L3 | L26 L25 L10 L9 | L14 L13 L24 L27 | L1 L2 L17 L24 L25 L18 | L18 L25 L24 L17
fillet "Сопряжение3" radius 0.2 4 edges at (4.55, 0, 2.5) (0, -4.66, 2.5) (0, 4.66, 2.5) (-4.55, 0, 2.5)
sketch "Эскиз6" plane through (0, 0, 2.5) normal (0, 0, 1) x (1, 0, 0)
  line L0 (3.85, -4.16) -> (-3.85, -4.16)
  line L1 (-4.05, -3.96) -> (-4.05, 3.96)
  line L2 (-3.85, 4.16) -> (3.85, 4.16)
  line L3 (4.05, 3.96) -> (4.05, -3.96)
  arc A0 (-4.05, -3.96) -> (-3.85, -4.16) centre (-3.85, -3.96) ccw
  arc A1 (3.85, -4.16) -> (4.05, -3.96) centre (3.85, -3.96) ccw
  arc A2 (4.05, 3.96) -> (3.85, 4.16) centre (3.85, 3.96) ccw
  arc A3 (-3.85, 4.16) -> (-4.05, 3.96) centre (-3.85, 3.96) ccw
  constraints: 8 end point, 8 point on circle, 8 tangent, 4 centre point, 3 equal radius, 2 parallel, 1 horizontal, 1 perpendicular
extrude "Выдавливание12" add sketch "Эскиз6" along normal blind 0.05
ref_plane "РабПлоскость3" through (0, 0, 2.55) normal (0, 0, 1) x (1, 0, 0)
sketch "Эскиз10" plane through (0, 0, 2.55) normal (0, 0, 1) x (1, 0, 0)
  line L0 (3.85, -4.16) -> (-3.85, -4.16)
  line L1 (-4.05, -3.96) -> (-4.05, 3.96)
  line L2 (-3.85, 4.16) -> (3.85, 4.16)
  line L3 (4.05, 3.96) -> (4.05, -3.96)
  arc A0 (-4.05, -3.96) -> (-3.85, -4.16) centre (-3.85, -3.96) ccw
  arc A1 (3.85, -4.16) -> (4.05, -3.96) centre (3.85, -3.96) ccw
  arc A2 (4.05, 3.96) -> (3.85, 4.16) centre (3.85, 3.96) ccw
  arc A3 (-3.85, 4.16) -> (-4.05, 3.96) centre (-3.85, 3.96) ccw
  line L4 (-4.05, 3.96) -> (-4.05, -3.96) projected
  line L5 (-4.05, 2.6625) -> (-2.5525, 4.16)
  line L6 (3.85, 4.16) -> (-3.85, 4.16) projected
  line L7 (-4.05, 2.6625) -> (-1.9322, 2.6625) construction
  dimension "d643" = 45
  constraints: 12 end point, 8 point on circle, 8 tangent, 4 centre point, 3 equal radius, 2 horizontal, 2 parallel, 2 point on line, 1 equal length, 1 perpendicular
  measures "d643" angle of L7 L5
extrude "Выдавливание13" add sketch "Эскиз10" along normal blind 0.001 contours L1 A3 L2 L5
sketch "Sketch11" plane through (0, 0, 0.01) normal (0, 0, -1) x (-1, 0, 0)
  line L0 (3.4589, 4.378) -> (3.0258, 4.128)
  line L1 (3.0258, 4.128) -> (3.0258, 4.628)
  line L2 (3.0258, 4.628) -> (3.4589, 4.378)
  point P0 (0, 0)
  point P1 (3.1702, 4.378)
  dimension "d639" = 0.5
  constraints: 6 end point, 1 horizontal alignment, 7 other
  measures "d639" distance of L0.end L1.end
extrude "Extrusion14" add sketch "Sketch11" along normal blind 0.001